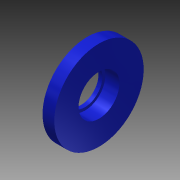
# Autodesk Inventor part: Small Bearing Cover
Saved by Autodesk Inventor 2014 (Build 180170000, 170)
## iProperties
Created: 2015-02-07
Part Number: Small Bearing Cover
Material: Generic
Document SubType Name: Modeling
Designer: Spooner
Density: 1 g/cm^3
Appearance: Blue - Wall Paint - Glossy
Author: Spooner
Autodesk Inventor part; units mm, degrees
ref_plane "YZ Plane" through (0, 0, 0) normal (1, 0, 0) x (0, 1, 0)
ref_plane "XZ Plane" through (0, 0, 0) normal (0, 1, 0) x (-1, 0, 0)
ref_plane "XY Plane" through (0, 0, 0) normal (0, 0, 1) x (1, 0, 0)
sketch "Sketch1" plane through (0, 0, 0) normal (0, 0, 1) x (1, 0, 0)
  line L0 (0, 13.0175) -> (10.16, 13.0175)
  line L1 (10.16, -13.0175) -> (10.16, 13.0175)
  line L2 (0, 13.0175) -> (0, -13.0175)
  line L3 (9.525, 16.8275) -> (24.13, 16.8275)
  line L4 (9.525, 20.6375) -> (9.525, 16.8275)
  line L5 (0.635, 16.8275) -> (0.635, 20.6375)
  line L6 (0.3356, 29.337) -> (9.8244, 29.337)
  line L7 (8.89, 29.083) -> (1.27, 29.083)
  line L8 (1.27, 29.083) -> (1.27, 14.2875)
  line L9 (8.89, 29.083) -> (8.89, 13.2715)
  line L10 (8.89, 13.2715) -> (-0.254, 13.2715)
  line L11 (-0.254, 13.2715) -> (-0.254, 11.3665)
  line L12 (-0.254, 11.3665) -> (-2.794, 11.3665)
  line L13 (-2.794, 11.3665) -> (-2.794, 14.2875)
  line L14 (-2.794, 14.2875) -> (1.27, 14.2875)
  line L15 (-13.97, 16.8275) -> (0.635, 16.8275)
  line L16 (31.75, 0) -> (-21.59, 0)
  point P0 (0, 0)
revolve "Revolution1" add sketch "Sketch1" angle 360 about axis through (5.16, 0, 0) along (-1, 0, 0) contours L9 L10 L11 L12 L13 L14 L8 L7
fillet "Fillet1" radius 3.175 1 edges at (1.27, -14.2875, 0)
equation "\"d1\" = d0"
equation "\"d4\" = d3"
equation "\"d0\" = 0.635"
equation "\"d3\" = 0.254"
body "Solid1"
